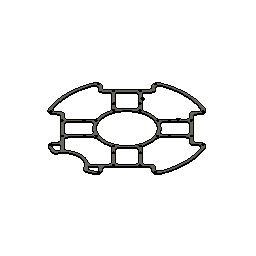
下板 v13 (Autodesk Fusion 360 design; units mm, degrees)
Autodesk Fusion 360 part; units mm, degrees
note: some values were not read from the file. Chosen so that the rebuilt part matches the saved one: which face or edge a step refers to; which pieces of a blend or face edit are solid. Set by a fixed rule: which sketch regions a step uses.
(part 1 of 5)
sketch "スケッチ1" plane through (0, 0, 0) normal (0, 0, 1) x (1, 0, 0)
  line L0 (-58.124, 63.7809) -> (-63.7809, 58.124)
  line L1 (-47.1639, 91.0045) -> (-40.8846, 84.7252)
  circle A0 centre (-62.3667, 62.3667) radius 1
  line L2 (-65.9022, 67.3164) -> (-70.852, 72.2662)
  line L3 (-35.8502, 54.9421) -> (-44.3355, 63.4273)
  arc A1 (-31.9886, 75.7742) -> (-31.9974, 82.8509) centre (-35.5257, 79.3082) ccw
  line L4 (-63.7809, 58.124) -> (-62.0978, 56.4409)
  line L5 (-33.8135, 84.7252) -> (-37.0951, 88.0068)
  line L6 (-68.0235, 65.1951) -> (-62.3667, 59.5382)
  line L7 (-54.5885, 60.2454) -> (-58.124, 63.7809)
  arc A2 (-46.9055, 91.138) -> (-47.1639, 91.0045) centre (0, 0) ccw
  arc A3 (-40.8846, 77.6541) -> (-40.8846, 84.7252) centre (-44.4201, 81.1896) ccw
  line L8 (-49.7234, 68.8153) -> (-68.8153, 49.7234)
  arc A4 (-84.7252, 40.8846) -> (-77.6541, 40.8846) centre (-81.1896, 44.4201) ccw
  line L9 (-55.6492, 27.3649) -> (-37.9715, 9.6872)
  arc A5 (-82.8374, 31.9257) -> (-75.8019, 31.9609) centre (-79.3374, 35.4964) ccw
  line L10 (-49.9923, 33.0217) -> (-53.8814, 36.9108)
  arc A6 (-88.0068, 37.0951) -> (-96.2368, 35.2806) centre (-91.5424, 33.5596) ccw
  line L11 (-31.9611, 14.9905) -> (-32.3146, 15.3441)
  circle A7 centre (-49.8155, 26.1275) radius 1.75
  line L12 (-34.167, -17.1965) -> (-34.0956, -17.125)
  arc A8 (-89.7814, 45.9408) -> (-97.869, 44.4738) centre (-93.3169, 42.4052) ccw
  line L13 (-83.0899, 32.1782) -> (-81.1896, 30.278)
  circle A9 centre (-39.2089, 15.5208) radius 1.75
  line L14 (-80.8769, 30.5907) -> (-81.1896, 30.278)
  line L15 (-85.4323, 41.5917) -> (-91.0045, 47.1639)
  line L16 (-86.1394, 35.2277) -> (-82.8374, 31.9257)
  line L17 (-88.4889, 37.5772) -> (-86.1394, 35.2277)
  line L18 (-85.4323, 41.5917) -> (-84.7252, 40.8846)
  line L19 (-70.852, 72.2662) -> (-72.2662, 70.852)
  arc A10 (-96.2368, 35.2806) -> (-96.2368, -35.2806) centre (0, 0) ccw
  line L20 (-49.7234, 68.8153) -> (-68.8153, 49.7234)
  arc A11 (-35.2806, 96.2368) -> (-37.0951, 88.0068) centre (-33.5596, 91.5424) ccw
  line L21 (-49.7234, 68.8153) -> (-40.8846, 77.6541)
  line L22 (-47.1639, 91.0045) -> (-45.9408, 89.7814)
  line L23 (-72.2662, 70.852) -> (-67.3164, 65.9022)
  arc A12 (-97.869, 44.4738) -> (-97.869, -44.4738) centre (0, 0) ccw
  circle A13 centre (-26.1275, 49.8155) radius 1.75
  line L24 (-59.5382, 62.3667) -> (-65.1951, 68.0235)
  line L25 (-36.9108, 53.8814) -> (-33.0217, 49.9923)
  line L26 (-37.5772, -88.4889) -> (-35.2277, -86.1394)
  arc A14 (-40.3326, -91.2443) -> (-39.6929, -94.5025) centre (-38.9184, -92.6585) ccw
  arc A15 (-37.9256, -100.5859) -> (-37.9262, -100.5876) centre (0, -113.3) ccw
  arc A16 (-31.321, -97.5974) -> (-31.2855, -97.6087) centre (0, 0) ccw
  line L27 (-84.7252, -33.8135) -> (-88.0068, -37.0951)
  line L28 (-41.5917, -85.4323) -> (-40.8846, -84.7252)
  arc A17 (-44.4738, -97.869) -> (-37.8014, -100.6345) centre (0, 0) ccw
  line L29 (-91.0045, -47.1639) -> (-85.4323, -41.5917)
  arc A18 (-39.6929, -94.5025) -> (-37.7434, -95.2979) centre (0, 0) ccw
  arc A19 (-40.8846, -84.7252) -> (-40.8846, -77.6541) centre (-44.4201, -81.1896) ccw
  arc A20 (-37.9256, -100.5859) -> (-37.9262, -100.5876) centre (0, -113.3) ccw
  arc A21 (-77.6541, -33.8135) -> (-84.7252, -33.8135) centre (-81.1896, -37.349) ccw
  line L30 (-41.5917, -85.4323) -> (-45.9408, -89.7814)
  line L31 (-91.0045, -47.1639) -> (-89.7814, -45.9408)
  arc A22 (-97.869, -44.4738) -> (-89.7814, -45.9408) centre (-93.3169, -42.4052) ccw
  circle A23 centre (-15.5208, 39.2089) radius 1.75
  line L32 (-65.1951, 68.0235) -> (-68.0235, 65.1951)
  line L33 (-69.0842, 69.0842) -> (-47.1639, 91.0045)
  line L34 (-15.3441, 32.3146) -> (-14.9905, 31.9611)
  line L35 (-91.0045, 47.1639) -> (-69.0842, 69.0842)
  line L36 (-37.9715, 9.6872) -> (-9.6872, 37.9715)
  line L37 (-27.3649, 55.6492) -> (-55.6492, 27.3649)
  line L38 (-63.4273, 44.3355) -> (-54.9421, 35.8502)
  line L39 (-62.0978, 56.4409) -> (-77.6541, 40.8846)
  arc A24 (0, 107.5) -> (-44.4738, 97.869) centre (0, 0) ccw
  line L40 (-56.4409, -62.0978) -> (-40.8846, -77.6541)
  line L41 (-54.9421, 35.8502) -> (-35.8502, 54.9421)
  arc A25 (-44.4738, 97.869) -> (-45.9408, 89.7814) centre (-42.4052, 93.3169) ccw
  line L42 (-14.9905, 31.9611) -> (-31.9611, 14.9905)
  line L43 (-9.6872, 37.9715) -> (-27.3649, 55.6492)
  arc A26 (0, 102.5) -> (-35.2806, 96.2368) centre (0, 0) ccw
  arc A27 (-77.6541, -40.8846) -> (-84.7252, -40.8846) centre (-81.1896, -44.4201) ccw
  arc A28 (-31.321, -97.5974) -> (-31.2855, -97.6087) centre (0, 0) ccw
  line L44 (-56.4409, -62.0978) -> (-62.0978, -56.4409)
  line L45 (-68.8153, -49.7234) -> (-49.7234, -68.8153)
  line L46 (-17.125, -34.0956) -> (-17.1965, -34.167)
  line L47 (-91.0045, -47.1639) -> (-84.7252, -40.8846)
  line L48 (-56.4409, -62.0978) -> (-62.0978, -56.4409)
  arc A29 (-32.3993, -86.1394) -> (-35.2277, -86.1394) centre (-33.8135, -87.5536) ccw
  line L49 (-68.8153, -49.7234) -> (-49.7234, -68.8153)
  line L50 (-68.8153, -49.7234) -> (-77.6541, -40.8846)
  line L51 (-32.3993, -86.1394) -> (-32.0426, -86.496)
  arc A30 (-37.9256, -100.5859) -> (-37.9262, -100.5876) centre (0, -113.3) ccw
  line L52 (-37.5772, -88.4889) -> (-40.3326, -91.2443)
  arc A31 (-96.2368, -35.2806) -> (-88.0068, -37.0951) centre (-91.5424, -33.5596) ccw
  arc A32 (-45.9408, -89.7814) -> (-44.4738, -97.869) centre (-42.4052, -93.3169) ccw
  arc A33 (-37.9256, -100.5859) -> (-37.8014, -100.6345) centre (-36.0432, -95.9538) ccw
  line L53 (-30.5907, -80.8769) -> (-21.5579, -89.9097)
  line L54 (-32.0426, -86.496) -> (-26.1835, -92.3551)
  line L55 (-37.7434, -95.2979) -> (-37.7266, -95.3045)
  line L56 (-23.7812, -100.8277) -> (-23.7402, -100.844)
  arc A34 (-43.0296, -15.8059) -> (-41.7301, -10.9963) centre (-46.5651, -12.2704) ccw
  arc A35 (-41.7301, 10.9963) -> (-41.7301, -10.9963) centre (0, 0) ccw
  line L57 (-62.6322, 42.4797) -> (-43.4926, 23.3401)
  arc A36 (-24.0851, 35.8083) -> (-35.8083, 24.0851) centre (0, 0) ccw
  arc A37 (-24.0851, 35.8083) -> (-35.8083, 24.0851) centre (0, 0) ccw
  arc A38 (0, 43.1547) -> (-10.9963, 41.7301) centre (0, 0) ccw
  arc A39 (0, 43.1547) -> (-10.9963, 41.7301) centre (0, 0) ccw
  arc A40 (-24.0851, 35.8083) -> (-35.8083, 24.0851) centre (0, 0) ccw
  arc A41 (-24.0851, 35.8083) -> (-23.3401, 43.4926) centre (-26.8756, 39.9571) ccw
  arc A42 (0, 43.1547) -> (-10.9963, 41.7301) centre (0, 0) ccw
  arc A43 (-24.0851, 35.8083) -> (-23.3401, 43.4926) centre (-26.8756, 39.9571) ccw
  arc A44 (-43.0296, -15.8059) -> (-41.7301, -10.9963) centre (-46.5651, -12.2704) ccw
  line L58 (-66.1678, 38.9441) -> (-43.0296, 15.8059)
  line L59 (-62.6322, 42.4797) -> (-43.4926, 23.3401)
  arc A45 (-41.7301, 10.9963) -> (-43.0296, 15.8059) centre (-46.5651, 12.2704) ccw
  line L60 (-66.1678, 38.9441) -> (-43.0296, 15.8059)
  arc A46 (-15.8059, 43.0296) -> (-10.9963, 41.7301) centre (-12.2704, 46.5651) ccw
  arc A47 (-15.8059, 43.0296) -> (-10.9963, 41.7301) centre (-12.2704, 46.5651) ccw
  arc A48 (-43.4926, 23.3401) -> (-35.8083, 24.0851) centre (-39.9571, 26.8756) ccw
  arc A49 (-43.4926, 23.3401) -> (-35.8083, 24.0851) centre (-39.9571, 26.8756) ccw
  arc A50 (-41.7301, 10.9963) -> (-41.7301, -10.9963) centre (0, 0) ccw
  arc A51 (-41.7301, 10.9963) -> (-41.7301, -10.9963) centre (0, 0) ccw
  arc A52 (-41.7301, 10.9963) -> (-43.0296, 15.8059) centre (-46.5651, 12.2704) ccw
  arc A53 (-10.9963, -41.7301) -> (-15.8059, -43.0296) centre (-12.2704, -46.5651) ccw
  line L61 (-38.9441, 66.1678) -> (-15.8059, 43.0296)
  arc A54 (-35.8083, -24.0851) -> (-24.0851, -35.8083) centre (0, 0) ccw
  arc A55 (-35.8083, -24.0851) -> (-43.4926, -23.3401) centre (-39.9571, -26.8756) ccw
  arc A56 (-10.9963, -41.7301) -> (-15.8059, -43.0296) centre (-12.2704, -46.5651) ccw
  line L62 (-42.4797, 62.6322) -> (-23.3401, 43.4926)
  line L63 (-42.4797, 62.6322) -> (-23.3401, 43.4926)
  arc A57 (-35.8083, -24.0851) -> (-24.0851, -35.8083) centre (0, 0) ccw
  line L64 (-62.6322, -42.4797) -> (-43.4926, -23.3401)
  arc A58 (-10.9963, -41.7301) -> (0, -43.1547) centre (0, 0) ccw
  arc A59 (-23.3401, -43.4926) -> (-24.0851, -35.8083) centre (-26.8756, -39.9571) ccw
  arc A60 (-10.9963, -41.7301) -> (0, -43.1547) centre (0, 0) ccw
  line L65 (-38.9441, 66.1678) -> (-15.8059, 43.0296)
  arc A61 (-35.8083, -24.0851) -> (-24.0851, -35.8083) centre (0, 0) ccw
  line L66 (-62.6322, -42.4797) -> (-43.4926, -23.3401)
  line L67 (-38.9441, -66.1678) -> (-15.8059, -43.0296)
  line L68 (-38.9441, -66.1678) -> (-29.7476, -56.9712)
  line L69 (-66.1678, -38.9441) -> (-43.0296, -15.8059)
  arc A62 (-29.5575, -103.3567) -> (-23.7528, -100.868) centre (-28.1827, -98.5494) ccw
  line L70 (-42.4797, -62.6322) -> (-23.3401, -43.4926)
  line L71 (-66.1678, -38.9441) -> (-43.0296, -15.8059)
  arc A63 (0, -86.4905) -> (-23.7528, -100.868) centre (0, -113.3) ccw
  arc A64 (-39.6929, -94.5025) -> (-32.0144, -97.3721) centre (0, 0) ccw
  arc A65 (-39.6929, -94.5025) -> (-32.0144, -97.3721) centre (0, 0) ccw
  arc A66 (-44.4738, -97.869) -> (-29.5575, -103.3567) centre (0, 0) ccw
  line L72 (-42.4797, -62.6322) -> (-23.3401, -43.4926)
  arc A67 (0, 38.1547) -> (0, -38.1547) centre (0, 0) ccw
  arc A68 (-44.4738, -97.869) -> (-29.5575, -103.3567) centre (0, 0) ccw
  arc A69 (-32.0144, -97.3721) -> (-26.3162, -95.431) centre (-30.4528, -92.6222) ccw
  arc A70 (0, -86.4905) -> (-23.7528, -100.868) centre (0, -113.3) ccw
  arc A71 (0, 38.1547) -> (0, -38.1547) centre (0, 0) ccw
  arc A72 (0, -81.4905) -> (-21.5579, -89.9097) centre (0, -113.3) ccw
  arc A73 (-25.9652, -94.9247) -> (-26.3162, -95.431) centre (0, -113.3) ccw
  arc A74 (0, -81.4905) -> (-21.5579, -89.9097) centre (0, -113.3) ccw
  arc A75 (-25.9652, -94.9247) -> (-26.3162, -95.431) centre (0, -113.3) ccw
  line L73 (-62.6322, 42.4797) -> (-63.9577, 43.8051)
  line L74 (-66.1678, 38.9441) -> (-67.4932, 40.2696)
  line L75 (-42.4797, 62.6322) -> (-43.8051, 63.9577)
  line L76 (-38.9441, 66.1678) -> (-40.2696, 67.4932)
  line L77 (-62.6322, -42.4797) -> (-65.8101, -45.6575)
  line L78 (-66.1678, -38.9441) -> (-69.3456, -42.122)
  line L79 (-42.4797, -62.6322) -> (-45.6575, -65.8101)
  line L80 (-38.9441, -66.1678) -> (-42.122, -69.3456)
  line L81 (-75.8019, 31.9609) -> (-67.4932, 40.2696)
  line L82 (-63.9577, 43.8051) -> (-43.8051, 63.9577)
  line L83 (-40.2696, 67.4932) -> (-31.9886, 75.7742)
  line L84 (-69.3456, -42.122) -> (-77.6541, -33.8135)
  line L85 (-30.5907, -80.8769) -> (-42.122, -69.3456)
  line L86 (-45.6575, -65.8101) -> (-65.8101, -45.6575)
  arc A76 (-25.9652, -94.9247) -> (-26.1835, -92.3551) centre (-27.5978, -93.7693) ccw
  circle A77 centre (-91.0045, 47.1639) radius 0.5
  arc A78 (0, 102.5) -> (0, -102.5) centre (0, 0) ccw
  line L87 (-17.1965, -34.167) -> (-17.4152, -33.9483)
  line L88 (-33.9483, -17.4152) -> (-34.167, -17.1965)
  line L89 (-17.1965, -34.167) -> (-17.4152, -33.9483)
  line L90 (-33.9483, -17.4152) -> (-34.167, -17.1965)
  line L91 (-17.1965, -34.167) -> (-17.4152, -33.9483)
  line L92 (-33.9483, -17.4152) -> (-34.167, -17.1965)
  line L93 (-69.0842, -69.0842) -> (-91.0045, -47.1639)
  line L94 (-47.1639, -91.0045) -> (-69.0842, -69.0842)
  line L95 (-67.3164, -65.9022) -> (-72.2662, -70.852)
  line L96 (-70.852, -72.2662) -> (-65.9022, -67.3164)
  line L97 (-72.2662, -70.852) -> (-70.852, -72.2662)
  line L98 (-68.0235, -65.1951) -> (-65.1951, -68.0235)
  line L99 (-62.3667, -59.5382) -> (-68.0235, -65.1951)
  line L100 (-65.1951, -68.0235) -> (-59.5382, -62.3667)
  circle A79 centre (-62.3667, -62.3667) radius 1
  line L101 (-63.7809, -58.124) -> (-58.124, -63.7809)
  line L102 (-58.124, -63.7809) -> (-56.4409, -62.0978)
  line L103 (-60.2454, -54.5885) -> (-63.7809, -58.124)
  line L104 (-44.3355, -63.4273) -> (-35.8502, -54.9421)
  line L105 (-54.9421, -35.8502) -> (-63.4273, -44.3355)
  line L106 (-35.8502, -54.9421) -> (-54.9421, -35.8502)
  line L107 (-53.8814, -36.9108) -> (-49.9923, -33.0217)
  line L108 (-33.0217, -49.9923) -> (-36.9108, -53.8814)
  line L109 (-55.6492, -27.3649) -> (-27.3649, -55.6492)
  circle A80 centre (-49.8155, -26.1275) radius 1.75
  circle A81 centre (-39.2089, -15.5208) radius 1.75
  circle A82 centre (-15.5208, -39.2089) radius 1.75
  circle A83 centre (-26.1275, -49.8155) radius 1.75
  line L110 (-27.3649, -55.6492) -> (-9.6872, -37.9715)
  line L111 (-9.6872, -37.9715) -> (-37.9715, -9.6872)
  line L112 (-31.9611, -14.9905) -> (-14.9905, -31.9611)
  line L113 (-37.9715, -9.6872) -> (-55.6492, -27.3649)
  line L114 (-14.9905, -31.9611) -> (-15.3441, -32.3146)
  line L115 (-32.3146, -15.3441) -> (-31.9611, -14.9905)
  arc A84 (0, -102.5) -> (0, 102.5) centre (0, 0) ccw
  line L116 (68.0235, -65.1951) -> (65.1951, -68.0235)
  line L117 (91.0045, -47.1639) -> (89.7814, -45.9408)
  arc A85 (41.7301, -10.9963) -> (41.7301, 10.9963) centre (0, 0) ccw
  line L118 (66.1678, -38.9441) -> (69.3456, -42.122)
  arc A86 (88.0068, -37.0951) -> (96.2368, -35.2806) centre (91.5424, -33.5596) ccw
  arc A87 (41.7301, -10.9963) -> (41.7301, 10.9963) centre (0, 0) ccw
  line L119 (69.3456, -42.122) -> (77.6541, -33.8135)
  arc A88 (84.7252, -40.8846) -> (77.6541, -40.8846) centre (81.1896, -44.4201) ccw
  line L120 (91.0045, -47.1639) -> (84.7252, -40.8846)
  line L121 (62.3667, -59.5382) -> (68.0235, -65.1951)
  line L122 (70.852, -72.2662) -> (65.9022, -67.3164)
  arc A89 (96.2368, -35.2806) -> (96.2368, 35.2806) centre (0, 0) ccw
  line L123 (65.1951, -68.0235) -> (59.5382, -62.3667)
  circle A90 centre (62.3667, -62.3667) radius 1
  line L124 (0, 107.5) -> (0, -102.5)
  line L125 (63.7809, -58.124) -> (58.124, -63.7809)
  line L126 (69.0842, -69.0842) -> (91.0045, -47.1639)
  line L127 (67.3164, -65.9022) -> (72.2662, -70.852)
  line L128 (58.124, -63.7809) -> (56.4409, -62.0978)
  line L129 (72.2662, -70.852) -> (70.852, -72.2662)
  line L130 (68.8153, -49.7234) -> (49.7234, -68.8153)
  line L131 (49.7234, 68.8153) -> (68.8153, 49.7234)
  line L132 (35.8502, -54.9421) -> (54.9421, -35.8502)
  line L133 (45.6575, -65.8101) -> (65.8101, -45.6575)
  arc A91 (10.9963, 41.7301) -> (0, 43.1547) centre (0, 0) ccw
  line L134 (56.4409, -62.0978) -> (40.8846, -77.6541)
  line L135 (66.1678, -38.9441) -> (43.0296, -15.8059)
  line L136 (62.6322, -42.4797) -> (43.4926, -23.3401)
  arc A92 (24.0851, -35.8083) -> (23.3401, -43.4926) centre (26.8756, -39.9571) ccw
  arc A93 (10.9963, 41.7301) -> (0, 43.1547) centre (0, 0) ccw
  arc A94 (35.2806, 96.2368) -> (0, 102.5) centre (0, 0) ccw
  arc A95 (15.8059, -43.0296) -> (10.9963, -41.7301) centre (12.2704, -46.5651) ccw
  line L137 (68.8153, -49.7234) -> (49.7234, -68.8153)
  line L138 (66.1678, -38.9441) -> (43.0296, -15.8059)
  line L139 (63.9577, 43.8051) -> (43.8051, 63.9577)
  arc A96 (0, -43.1547) -> (10.9963, -41.7301) centre (0, 0) ccw
  line L140 (91.0045, 47.1639) -> (69.0842, 69.0842)
  arc A97 (15.8059, -43.0296) -> (10.9963, -41.7301) centre (12.2704, -46.5651) ccw
  arc A98 (10.9963, 41.7301) -> (0, 43.1547) centre (0, 0) ccw
  line L141 (42.4797, 62.6322) -> (23.3401, 43.4926)
  arc A99 (0, -43.1547) -> (10.9963, -41.7301) centre (0, 0) ccw
  arc A100 (44.4738, 97.869) -> (0, 107.5) centre (0, 0) ccw
  line L142 (62.6322, -42.4797) -> (43.4926, -23.3401)
  line L143 (27.3649, -55.6492) -> (9.6872, -37.9715)
  line L144 (62.0978, 56.4409) -> (77.6541, 40.8846)
  line L145 (54.9421, 35.8502) -> (35.8502, 54.9421)
  line L146 (38.9441, 66.1678) -> (15.8059, 43.0296)
  circle A101 centre (26.1275, 49.8155) radius 1.75
  line L147 (49.7234, 68.8153) -> (68.8153, 49.7234)
  circle A102 centre (26.1275, -49.8155) radius 1.75
  arc A103 (97.869, -44.4738) -> (97.869, 44.4738) centre (0, 0) ccw
  line L148 (33.0217, -49.9923) -> (36.9108, -53.8814)
  circle A104 centre (15.5208, -39.2089) radius 1.75
  line L149 (54.9421, -35.8502) -> (63.4273, -44.3355)
  line L150 (68.8153, -49.7234) -> (77.6541, -40.8846)
  line L151 (60.2454, -54.5885) -> (63.7809, -58.124)
  line L152 (56.4409, -62.0978) -> (62.0978, -56.4409)
  line L153 (56.4409, -62.0978) -> (62.0978, -56.4409)
  arc A105 (41.7301, -10.9963) -> (41.7301, 10.9963) centre (0, 0) ccw
  arc A106 (89.7814, -45.9408) -> (97.869, -44.4738) centre (93.3169, -42.4052) ccw
  line L154 (84.7252, -33.8135) -> (88.0068, -37.0951)
  line L155 (91.0045, -47.1639) -> (85.4323, -41.5917)
  arc A107 (84.7252, -33.8135) -> (77.6541, -33.8135) centre (81.1896, -37.349) ccw
  arc A108 (0, -38.1547) -> (0, 38.1547) centre (0, 0) ccw
  line L156 (62.6322, -42.4797) -> (65.8101, -45.6575)
  line L157 (42.4797, 62.6322) -> (23.3401, 43.4926)
  line L158 (36.9108, 53.8814) -> (33.0217, 49.9923)
  line L159 (75.8019, 31.9609) -> (67.4932, 40.2696)
  line L160 (17.1965, -34.167) -> (17.4152, -33.9483)
  line L161 (53.8814, -36.9108) -> (49.9923, -33.0217)
  arc A109 (24.0851, -35.8083) -> (35.8083, -24.0851) centre (0, 0) ccw
  line L162 (17.1965, -34.167) -> (17.4152, -33.9483)
  line L163 (85.4323, 41.5917) -> (91.0045, 47.1639)
  line L164 (38.9441, 66.1678) -> (40.2696, 67.4932)
  line L165 (55.6492, -27.3649) -> (27.3649, -55.6492)
  line L166 (27.3649, 55.6492) -> (55.6492, 27.3649)
  line L167 (42.4797, -62.6322) -> (23.3401, -43.4926)
  line L168 (66.1678, 38.9441) -> (43.0296, 15.8059)
  line L169 (38.9441, 66.1678) -> (15.8059, 43.0296)
  line L170 (32.3146, -15.3441) -> (31.9611, -14.9905)
  line L171 (33.9483, -17.4152) -> (34.167, -17.1965)
  line L172 (55.6492, 27.3649) -> (37.9715, 9.6872)
  line L173 (33.9483, -17.4152) -> (34.167, -17.1965)
  line L174 (17.1965, -34.167) -> (17.4152, -33.9483)
  line L175 (40.2696, 67.4932) -> (31.9886, 75.7742)
  arc A110 (24.0851, -35.8083) -> (35.8083, -24.0851) centre (0, 0) ccw
  line L176 (35.8502, 54.9421) -> (44.3355, 63.4273)
  line L177 (62.6322, 42.4797) -> (43.4926, 23.3401)
  line L178 (62.6322, 42.4797) -> (43.4926, 23.3401)
  circle A111 centre (39.2089, 15.5208) radius 1.75
  line L179 (85.4323, 41.5917) -> (84.7252, 40.8846)
  line L180 (34.167, -17.1965) -> (34.0956, -17.125)
  line L181 (54.5885, 60.2454) -> (58.124, 63.7809)
  line L182 (37.9715, -9.6872) -> (55.6492, -27.3649)
  line L183 (47.1639, -91.0045) -> (69.0842, -69.0842)
  circle A112 centre (49.8155, -26.1275) radius 1.75
  line L184 (14.9905, -31.9611) -> (15.3441, -32.3146)
  line L185 (38.9441, -66.1678) -> (15.8059, -43.0296)
  line L186 (9.6872, 37.9715) -> (27.3649, 55.6492)
  arc A113 (96.2368, 35.2806) -> (88.0068, 37.0951) centre (91.5424, 33.5596) ccw
  arc A114 (23.7528, -100.868) -> (29.5575, -103.3567) centre (28.1827, -98.5494) ccw
  line L187 (86.1394, 35.2277) -> (82.8374, 31.9257)
  line L188 (49.9923, 33.0217) -> (53.8814, 36.9108)
  line L189 (38.9441, -66.1678) -> (29.7476, -56.9712)
  line L190 (42.4797, -62.6322) -> (23.3401, -43.4926)
  arc A115 (24.0851, -35.8083) -> (35.8083, -24.0851) centre (0, 0) ccw
  circle A116 centre (39.2089, -15.5208) radius 1.75
  line L191 (31.9611, -14.9905) -> (14.9905, -31.9611)
  line L192 (62.6322, 42.4797) -> (63.9577, 43.8051)
  line L193 (49.7234, 68.8153) -> (40.8846, 77.6541)
  line L194 (83.0899, 32.1782) -> (81.1896, 30.278)
  line L195 (44.3355, -63.4273) -> (35.8502, -54.9421)
  line L196 (66.1678, 38.9441) -> (43.0296, 15.8059)
  arc A117 (35.8083, 24.0851) -> (43.4926, 23.3401) centre (39.9571, 26.8756) ccw
  line L197 (30.5907, -80.8769) -> (21.5579, -89.9097)
  line L198 (9.6872, -37.9715) -> (37.9715, -9.6872)
  line L199 (15.3441, 32.3146) -> (14.9905, 31.9611)
  line L200 (88.4889, 37.5772) -> (86.1394, 35.2277)
  line L201 (17.125, -34.0956) -> (17.1965, -34.167)
  arc A118 (41.7301, -10.9963) -> (43.0296, -15.8059) centre (46.5651, -12.2704) ccw
  line L202 (80.8769, 30.5907) -> (81.1896, 30.278)
  arc A119 (26.3162, -95.431) -> (32.0144, -97.3721) centre (30.4528, -92.6222) ccw
  line L203 (32.0426, -86.496) -> (26.1835, -92.3551)
  circle A120 centre (91.0045, 47.1639) radius 0.5
  arc A121 (77.6541, 40.8846) -> (84.7252, 40.8846) centre (81.1896, 44.4201) ccw
  line L204 (63.7809, 58.124) -> (62.0978, 56.4409)
  circle A122 centre (49.8155, 26.1275) radius 1.75
  line L205 (66.1678, 38.9441) -> (67.4932, 40.2696)
  arc A123 (43.0296, 15.8059) -> (41.7301, 10.9963) centre (46.5651, 12.2704) ccw
  line L206 (65.1951, 68.0235) -> (68.0235, 65.1951)
  arc A124 (29.5575, -103.3567) -> (44.4738, -97.869) centre (0, 0) ccw
  line L207 (47.1639, 91.0045) -> (40.8846, 84.7252)
  line L208 (37.5772, -88.4889) -> (35.2277, -86.1394)
  arc A125 (35.8083, 24.0851) -> (24.0851, 35.8083) centre (0, 0) ccw
  arc A126 (37.8014, -100.6345) -> (44.4738, -97.869) centre (0, 0) ccw
  arc A127 (10.9963, 41.7301) -> (15.8059, 43.0296) centre (12.2704, 46.5651) ccw
  arc A128 (23.7528, -100.868) -> (0, -86.4905) centre (0, -113.3) ccw
  arc A129 (10.9963, 41.7301) -> (15.8059, 43.0296) centre (12.2704, 46.5651) ccw
  arc A130 (75.8019, 31.9609) -> (82.8374, 31.9257) centre (79.3374, 35.4964) ccw
  arc A131 (43.0296, 15.8059) -> (41.7301, 10.9963) centre (46.5651, 12.2704) ccw
  arc A132 (23.3401, 43.4926) -> (24.0851, 35.8083) centre (26.8756, 39.9571) ccw
  arc A133 (32.0144, -97.3721) -> (39.6929, -94.5025) centre (0, 0) ccw
  line L209 (33.9483, -17.4152) -> (34.167, -17.1965)
  arc A134 (41.7301, -10.9963) -> (43.0296, -15.8059) centre (46.5651, -12.2704) ccw
  line L210 (69.0842, 69.0842) -> (47.1639, 91.0045)
  line L211 (23.7812, -100.8277) -> (23.7402, -100.844)
  arc A135 (35.8083, 24.0851) -> (24.0851, 35.8083) centre (0, 0) ccw
  arc A136 (40.8846, 84.7252) -> (40.8846, 77.6541) centre (44.4201, 81.1896) ccw
  arc A137 (45.9408, 89.7814) -> (44.4738, 97.869) centre (42.4052, 93.3169) ccw
  arc A138 (31.2855, -97.6087) -> (31.321, -97.5974) centre (0, 0) ccw
  line L212 (68.0235, 65.1951) -> (62.3667, 59.5382)
  line L213 (41.5917, -85.4323) -> (40.8846, -84.7252)
  arc A139 (23.7528, -100.868) -> (0, -86.4905) centre (0, -113.3) ccw
  line L214 (31.9611, 14.9905) -> (32.3146, 15.3441)
  arc A140 (37.9262, -100.5876) -> (37.9256, -100.5859) centre (0, -113.3) ccw
  circle A141 centre (15.5208, 39.2089) radius 1.75
  line L215 (30.5907, -80.8769) -> (42.122, -69.3456)
  arc A142 (21.5579, -89.9097) -> (0, -81.4905) centre (0, -113.3) ccw
  line L216 (14.9905, 31.9611) -> (31.9611, 14.9905)
  line L217 (41.5917, -85.4323) -> (45.9408, -89.7814)
  arc A143 (43.4926, -23.3401) -> (35.8083, -24.0851) centre (39.9571, -26.8756) ccw
  arc A144 (35.8083, 24.0851) -> (24.0851, 35.8083) centre (0, 0) ccw
  arc A145 (97.869, 44.4738) -> (89.7814, 45.9408) centre (93.3169, 42.4052) ccw
  line L218 (63.4273, 44.3355) -> (54.9421, 35.8502)
  arc A146 (35.2277, -86.1394) -> (32.3993, -86.1394) centre (33.8135, -87.5536) ccw
  line L219 (65.9022, 67.3164) -> (70.852, 72.2662)
  arc A147 (21.5579, -89.9097) -> (0, -81.4905) centre (0, -113.3) ccw
  line L220 (42.4797, 62.6322) -> (43.8051, 63.9577)
  arc A148 (31.9974, 82.8509) -> (31.9886, 75.7742) centre (35.5257, 79.3082) ccw
  line L221 (32.3993, -86.1394) -> (32.0426, -86.496)
  line L222 (72.2662, 70.852) -> (67.3164, 65.9022)
  arc A149 (29.5575, -103.3567) -> (44.4738, -97.869) centre (0, 0) ccw
  arc A150 (23.3401, 43.4926) -> (24.0851, 35.8083) centre (26.8756, 39.9571) ccw
  arc A151 (47.1639, 91.0045) -> (46.9055, 91.138) centre (0, 0) ccw
  arc A152 (39.6929, -94.5025) -> (40.3326, -91.2443) centre (38.9184, -92.6585) ccw
  arc A153 (35.8083, 24.0851) -> (43.4926, 23.3401) centre (39.9571, 26.8756) ccw
  line L223 (37.9715, 9.6872) -> (9.6872, 37.9715)
  arc A154 (37.9262, -100.5876) -> (37.9256, -100.5859) centre (0, -113.3) ccw
  arc A155 (26.1835, -92.3551) -> (25.9652, -94.9247) centre (27.5978, -93.7693) ccw
  arc A156 (37.8014, -100.6345) -> (37.9256, -100.5859) centre (36.0432, -95.9538) ccw
  line L224 (47.1639, 91.0045) -> (45.9408, 89.7814)
  line L225 (70.852, 72.2662) -> (72.2662, 70.852)
  arc A157 (37.9262, -100.5876) -> (37.9256, -100.5859) centre (0, -113.3) ccw
  line L226 (58.124, 63.7809) -> (63.7809, 58.124)
  line L227 (42.4797, -62.6322) -> (45.6575, -65.8101)
  circle A158 centre (62.3667, 62.3667) radius 1
  line L228 (37.7434, -95.2979) -> (37.7266, -95.3045)
  arc A159 (40.8846, -77.6541) -> (40.8846, -84.7252) centre (44.4201, -81.1896) ccw
  arc A160 (37.7434, -95.2979) -> (39.6929, -94.5025) centre (0, 0) ccw
  arc A161 (26.3162, -95.431) -> (25.9652, -94.9247) centre (0, -113.3) ccw
  arc A162 (37.0951, 88.0068) -> (35.2806, 96.2368) centre (33.5596, 91.5424) ccw
  arc A163 (26.3162, -95.431) -> (25.9652, -94.9247) centre (0, -113.3) ccw
  arc A164 (32.0144, -97.3721) -> (39.6929, -94.5025) centre (0, 0) ccw
  arc A165 (31.2855, -97.6087) -> (31.321, -97.5974) centre (0, 0) ccw
  line L229 (59.5382, 62.3667) -> (65.1951, 68.0235)
  line L230 (33.8135, 84.7252) -> (37.0951, 88.0068)
  arc A166 (44.4738, -97.869) -> (45.9408, -89.7814) centre (42.4052, -93.3169) ccw
  line L231 (38.9441, -66.1678) -> (42.122, -69.3456)
  line L232 (37.5772, -88.4889) -> (40.3326, -91.2443)
  arc A167 (0, -38.1547) -> (0, 38.1547) centre (0, 0) ccw
  line L233 (0, 107.5) -> (0, -86.4905)
  line L234 (-33.8135, 84.7252) -> (-31.9974, 82.8509)
  line L235 (33.8135, 84.7252) -> (31.9974, 82.8509)
  point P0 (-63.8655, -63.8655)
  point P1 (-81.1896, -37.349)
  point P2 (-63.8655, -63.8655)
  point P3 (-63.8655, -63.8655)
  point P4 (-37.349, 81.1896)
  point P5 (-12.2704, -46.5651)
  point P6 (-12.2704, 46.5651)
  point P7 (12.2704, -46.5651)
  point P8 (12.2704, 46.5651)
  point P9 (63.8655, -63.8655)
  point P10 (63.8655, -63.8655)
  point P11 (63.8655, -63.8655)
  point P12 (81.1896, -37.349)
  point P13 (12.2704, -46.5651)
  point P14 (37.349, 81.1896)
  point P15 (12.2704, 46.5651)
  point P16 (-12.2704, -46.5651)
  point P17 (-12.2704, 46.5651)
  dimension "d45" = 5
  dimension "d46" = 5
  dimension "d47" = 2
  dimension "d52" = 1
  constraint parallel L53 L85
  constraint tangent A18 L55
  constraint parallel L55 L56
  constraint coincident L58.end A45.end
  constraint coincident A46.start A47.start
  constraint coincident A34.start A44.start
  constraint coincident A53.end A56.end
  constraint coincident L57.end L59.end
  constraint coincident A41.end A43.end
  constraint coincident A55.end L64.end
  constraint coincident A59.start L70.end
  constraint coincident L58.end A45
  constraint coincident L57.end A48
  constraint coincident A41.end A43
  constraint coincident A47.start A46
  constraint coincident L58.end A52
  constraint coincident L57.end A49
  constraint coincident A43.end A41
  constraint coincident A46.start A47
  constraint tangent A69 A72
  constraint tangent A62 A70
  constraint concentric A36 A67
  constraint coincident A53.start A36
  constraint concentric A36 A50
  constraint concentric A50 A57
  constraint concentric A57 A58
  constraint coincident A63 L56.end
  constraint coincident A64 L55.end
  constraint concentric A72 A73
  constraint concentric A74 A75
  constraint perpendicular L73 L81
  constraint perpendicular L74 L81
  constraint perpendicular L75 L81
  constraint perpendicular L76 L81
  constraint perpendicular L77 L85
  constraint perpendicular L78 L85
  constraint perpendicular L79 L85
  constraint perpendicular L80 L85
  constraint collinear L81 L82
  constraint collinear L82 L83
  constraint collinear L84 L85
  constraint coincident L79.end L85
  constraint collinear L85 L86
  constraint coincident L82 L38.start
  constraint coincident L82 L3.end
  constraint tangent L54 A76
  constraint tangent A75 A76
  constraint coincident L15 L35.start
  constraint coincident L15.end A78
  constraint coincident A67 L87.end
  constraint coincident A67 L88.start
  constraint collinear L87 L88
  constraint collinear L89 L90
  constraint collinear L91 L92
  constraint coincident A67 L12.end
  constraint coincident A67 L46.start
  constraint coincident A78 L29.start
  measures "d45" radius of A69
  measures "d46" radius of A62
  measures "d47" radius of A76
  measures "d52" diameter of A77
extrude "押し出し1" add sketch "スケッチ1" along normal blind 1.5 contours L36 L43 A38 A39 A42 A46 A47 A67 A71 L124 L233 | L9 L36 L37 L43 L57 A36 A37 A40 A41 A43 L58 L59 A45 L60 A46 A47 A48 A49 A52 L61 L62 L63 L65 A67 A71 | A53 A56 A58 A60 A67 A71 L110 L111 L124 L233 | L9 L36 A34 A35 A44 A45 A50 A51 A52 A67 A71 L111 L113 | L12 L46 A34 A44 A53 A54 A55 A56 A57 L64 A59 A61 L66 L67 L69 L70 L71 L72 A67 A71 L87 L88 L89 L90 L91 L92 L109 L110 L111 L113 | A80 | A81 | A82 | A83 makes body 1
fillet "フィレット1" [no effect]
extrude "押し出し2" add sketch "スケッチ1" along normal blind 1.5 contours A24 A25 A26 A78 L124 L233 | A8 A10 A12 A22 A77 A78 | A84 L124 A94 A100 A137 L233 | L124 A91 A93 A98 A108 L186 A127 A129 L223 A167 L233 | L26 A14 A15 L27 L28 L29 A19 A20 A21 L30 A22 L40 A27 L44 L45 L47 L48 A29 L49 L50 L51 A30 L52 A31 A32 L53 L54 L64 L66 L67 L68 L69 L70 L71 L72 L77 L78 L79 L80 L84 L85 L86 A78 L109 A140 A154 A157 | L124 A95 A96 A97 A99 L143 A108 L198 A167 L233 | L141 L146 A108 L157 L166 L168 L169 L172 L177 L178 L186 L196 A117 A123 A125 A127 A129 A131 A132 A135 A144 A150 A153 L223 A167 | L135 L136 A92 A95 L138 A97 L142 L143 A108 L160 A109 L162 L165 L167 L171 L173 L174 A110 L180 L182 L185 L190 A115 L198 L201 A118 L209 A134 A143 A167 | A85 A87 A105 A108 L172 L182 L198 A118 A123 A131 A134 L223 A167 | A15 A17 A18 A20 A30 A32 L55 A64 A65 A66 A68 A78 A140 A154 A157 | A84 A89 A103 A106 A120 A145 | A15 A20 A30 A84 L118 A86 L119 A88 L120 L130 L133 L134 L135 L136 L137 L138 L142 L150 L152 L153 A106 L154 L155 A107 L156 L165 L167 L185 L189 L190 L197 L203 L208 L213 A140 L215 L217 A146 L221 A152 A154 A157 L227 A159 A166 L231 L232 | A15 A20 A30 A84 L124 L197 A119 L203 A128 A138 A139 A140 A142 A147 A154 A155 A157 A161 A163 A165 L233 | A15 A16 A20 A28 A30 L53 L54 A63 A69 A70 A72 A73 A74 A75 A76 A78 L124 A140 A154 A157 L233 | A15 A16 A17 A20 A28 A30 A33 A62 A63 A64 A65 A66 A68 A70 A78 A140 A154 A157 | A15 A20 A30 A84 A124 A126 A133 A140 A149 A154 A157 L228 A160 A164 A166 | A15 A20 A30 A84 A114 A124 A126 A128 A133 A138 A139 A140 A149 A154 A156 A157 A164 A165 bodies 1 makes body 2 at (0, 104.0092, 0)
extrude "押し出し3" add sketch "スケッチ1" along normal blind 1.5 contours L1 A1 L5 A3 L8 A4 A5 A6 A8 L13 L15 L16 L17 L18 L20 A11 L21 L37 L39 A25 L57 L58 L59 L60 L61 L62 L63 L65 L73 L74 L75 L76 L81 L82 L83 A77 A78 L234 | A84 L131 L139 L141 L144 L146 L147 L157 L159 L163 L164 L166 L168 L169 L175 L177 L178 L179 A113 L187 L192 L193 L194 L196 L200 A120 A121 L205 L207 A130 A136 A137 A145 L220 A148 A162 L230 L235 bodies 1 2
fillet "フィレット2" radius 5 16 edges at (40.2696, 67.4932, 0.75) (-40.2696, 67.4932, 0.75) (-43.8051, 63.9577, 0.75) (-63.9577, 43.8051, 0.75) (-67.4932, 40.2696, 0.75) (-69.3456, -42.122, 0.75) (-65.8101, -45.6575, 0.75) (-45.6575, -65.8101, 0.75) (-42.122, -69.3456, 0.75) (-21.5579, -89.9097, 0.75) (21.5579, -89.9097, 0.75) (42.122, -69.3456, 0.75) (45.6575, -65.8101, 0.75) (69.3456, -42.122, 0.75) (65.8101, -45.6575, 0.75) (67.4932, 40.2696, 0.75) on bodies 1
extrude "押し出し4" cut sketch "スケッチ1" along normal blind 100 contours A80 | A81 | A82 | A83 bodies 1
sketch "スケッチ2" plane through (0, 0, 0) normal (0, 0, -1) x (1, 0, 0)
  circle A0 centre (-26.1275, 49.8155) radius 1.75
  circle A1 centre (-39.2089, 15.5208) radius 1.75
  circle A2 centre (-15.5208, 39.2089) radius 1.75
  circle A3 centre (-49.8155, 26.1275) radius 1.75
  line L0 (-38.9441, -66.1678) -> (-15.8059, -43.0296)
  arc A4 (-10.9963, -41.7301) -> (-15.8059, -43.0296) centre (-12.2704, -46.5651) ccw
  arc A5 (-10.9963, -41.7301) -> (10.9963, -41.7301) centre (0, 0) ccw
  arc A6 (15.8059, -43.0296) -> (10.9963, -41.7301) centre (12.2704, -46.5651) ccw
  line L1 (15.8059, -43.0296) -> (38.9441, -66.1678)
  arc A7 (37.51, -70.2528) -> (38.9441, -66.1678) centre (33.9744, -66.7173) ccw
  line L2 (37.51, -70.2528) -> (31.9886, -75.7742)
  arc A8 (31.9886, -75.7742) -> (31.9974, -82.8509) centre (35.5257, -79.3082) ccw
  line L3 (31.9974, -82.8509) -> (33.8135, -84.7252)
  line L4 (33.8135, -84.7252) -> (37.0951, -88.0068)
  arc A9 (35.2806, -96.2368) -> (37.0951, -88.0068) centre (33.5596, -91.5424) ccw
  arc A10 (-35.2806, -96.2368) -> (35.2806, -96.2368) centre (0, 0) ccw
  arc A11 (-37.0951, -88.0068) -> (-35.2806, -96.2368) centre (-33.5596, -91.5424) ccw
  line L5 (-37.0951, -88.0068) -> (-33.8135, -84.7252)
  line L6 (-33.8135, -84.7252) -> (-31.9974, -82.8509)
  arc A12 (-31.9974, -82.8509) -> (-31.9886, -75.7742) centre (-35.5257, -79.3082) ccw
  line L7 (-31.9886, -75.7742) -> (-37.51, -70.2528)
  arc A13 (-38.9441, -66.1678) -> (-37.51, -70.2528) centre (-33.9744, -66.7173) ccw
  line L8 (-23.3401, -43.4926) -> (-42.4797, -62.6322)
  arc A14 (-46.5647, -61.198) -> (-42.4797, -62.6322) centre (-43.0292, -57.6625) ccw
  line L9 (-46.5647, -61.198) -> (-60.4221, -47.3407)
  arc A15 (-60.4221, -40.2696) -> (-60.4221, -47.3407) centre (-56.8866, -43.8051) ccw
  line L10 (-60.4221, -40.2696) -> (-43.4926, -23.3401)
  arc A16 (-35.8083, -24.0851) -> (-43.4926, -23.3401) centre (-39.9571, -26.8756) ccw
  arc A17 (-35.8083, -24.0851) -> (-24.0851, -35.8083) centre (0, 0) ccw
  arc A18 (-23.3401, -43.4926) -> (-24.0851, -35.8083) centre (-26.8756, -39.9571) ccw
  line L11 (-43.0296, -15.8059) -> (-63.9577, -36.7341)
  arc A19 (-71.0287, -36.7341) -> (-63.9577, -36.7341) centre (-67.4932, -33.1985) ccw
  line L12 (-71.0287, -36.7341) -> (-75.8019, -31.9609)
  arc A20 (-75.8019, -31.9609) -> (-82.8374, -31.9257) centre (-79.3374, -35.4964) ccw
  line L13 (-82.8374, -31.9257) -> (-88.0068, -37.0951)
  arc A21 (-96.2368, -35.2806) -> (-88.0068, -37.0951) centre (-91.5424, -33.5596) ccw
  arc A22 (-96.2368, 35.2806) -> (-96.2368, -35.2806) centre (0, 0) ccw
  arc A23 (-88.0068, 37.0951) -> (-96.2368, 35.2806) centre (-91.5424, 33.5596) ccw
  line L14 (-88.0068, 37.0951) -> (-84.7252, 33.8135)
  arc A24 (-84.7252, 33.8135) -> (-77.6541, 33.8135) centre (-81.1896, 37.349) ccw
  line L15 (-77.6541, 33.8135) -> (-72.863, 38.6046)
  arc A25 (-66.1678, 38.9441) -> (-72.863, 38.6046) centre (-69.3275, 35.0691) ccw
  line L16 (-66.1678, 38.9441) -> (-43.0296, 15.8059)
  arc A26 (-41.7301, 10.9963) -> (-43.0296, 15.8059) centre (-46.5651, 12.2704) ccw
  arc A27 (-41.7301, 10.9963) -> (-41.7301, -10.9963) centre (0, 0) ccw
  arc A28 (-43.0296, -15.8059) -> (-41.7301, -10.9963) centre (-46.5651, -12.2704) ccw
  arc A29 (-90.783, -46.7156) -> (-91.4938, -47.061) centre (-91.0045, -47.1639) ccw
  arc A30 (-90.783, -46.7156) -> (-89.7814, -45.9408) centre (-93.3169, -42.4052) ccw
  line L17 (-89.7814, -45.9408) -> (-84.7252, -40.8846)
  arc A31 (-77.6541, -40.8846) -> (-84.7252, -40.8846) centre (-81.1896, -44.4201) ccw
  line L18 (-77.6541, -40.8846) -> (-40.8846, -77.6541)
  arc A32 (-40.8846, -84.7252) -> (-40.8846, -77.6541) centre (-44.4201, -81.1896) ccw
  line L19 (-40.8846, -84.7252) -> (-45.9408, -89.7814)
  arc A33 (-45.9408, -89.7814) -> (-44.4738, -97.869) centre (-42.4052, -93.3169) ccw
  arc A34 (-44.4738, -97.869) -> (44.4738, -97.869) centre (0, 0) ccw
  arc A35 (44.4738, -97.869) -> (45.9408, -89.7814) centre (42.4052, -93.3169) ccw
  line L20 (45.9408, -89.7814) -> (40.8846, -84.7252)
  arc A36 (40.8846, -77.6541) -> (40.8846, -84.7252) centre (44.4201, -81.1896) ccw
  line L21 (40.8846, -77.6541) -> (77.6541, -40.8846)
  arc A37 (84.7252, -40.8846) -> (77.6541, -40.8846) centre (81.1896, -44.4201) ccw
  line L22 (84.7252, -40.8846) -> (89.7814, -45.9408)
  arc A38 (89.7814, -45.9408) -> (90.783, -46.7156) centre (93.3169, -42.4052) ccw
  arc A39 (91.4938, -47.061) -> (90.783, -46.7156) centre (91.0045, -47.1639) ccw
  arc A40 (91.4938, -47.061) -> (97.869, -44.4738) centre (93.3169, -42.4052) ccw
  arc A41 (97.869, -44.4738) -> (97.869, 44.4738) centre (0, 0) ccw
  arc A42 (97.869, 44.4738) -> (89.7814, 45.9408) centre (93.3169, 42.4052) ccw
  line L23 (89.7814, 45.9408) -> (84.7252, 40.8846)
  arc A43 (77.6541, 40.8846) -> (84.7252, 40.8846) centre (81.1896, 44.4201) ccw
  line L24 (77.6541, 40.8846) -> (40.8846, 77.6541)
  arc A44 (40.8846, 84.7252) -> (40.8846, 77.6541) centre (44.4201, 81.1896) ccw
  line L25 (40.8846, 84.7252) -> (45.9408, 89.7814)
  arc A45 (45.9408, 89.7814) -> (44.4738, 97.869) centre (42.4052, 93.3169) ccw
  arc A46 (44.4738, 97.869) -> (37.9262, 100.5876) centre (0, 0) ccw
  arc A47 (37.9256, 100.5859) -> (37.9262, 100.5876) centre (0, 113.3) ccw
  arc A48 (37.9256, 100.5859) -> (37.8014, 100.6345) centre (36.0432, 95.9538) ccw
  arc A49 (37.8014, 100.6345) -> (29.5575, 103.3567) centre (0, 0) ccw
  arc A50 (29.5575, 103.3567) -> (23.7528, 100.868) centre (28.1827, 98.5494) ccw
  arc A51 (-23.7528, 100.868) -> (23.7528, 100.868) centre (0, 113.3) ccw
  arc A52 (-23.7528, 100.868) -> (-29.5575, 103.3567) centre (-28.1827, 98.5494) ccw
  arc A53 (-29.5575, 103.3567) -> (-37.8014, 100.6345) centre (0, 0) ccw
  arc A54 (-37.8014, 100.6345) -> (-37.9256, 100.5859) centre (-36.0432, 95.9538) ccw
  arc A55 (-37.9262, 100.5876) -> (-37.9256, 100.5859) centre (0, 113.3) ccw
  arc A56 (-37.9262, 100.5876) -> (-44.4738, 97.869) centre (0, 0) ccw
  arc A57 (-44.4738, 97.869) -> (-45.9408, 89.7814) centre (-42.4052, 93.3169) ccw
  line L26 (-45.9408, 89.7814) -> (-40.8846, 84.7252)
  arc A58 (-40.8846, 77.6541) -> (-40.8846, 84.7252) centre (-44.4201, 81.1896) ccw
  line L27 (-40.8846, 77.6541) -> (-77.6541, 40.8846)
  arc A59 (-84.7252, 40.8846) -> (-77.6541, 40.8846) centre (-81.1896, 44.4201) ccw
  line L28 (-84.7252, 40.8846) -> (-89.7814, 45.9408)
  arc A60 (-89.7814, 45.9408) -> (-97.869, 44.4738) centre (-93.3169, 42.4052) ccw
  arc A61 (-97.869, 44.4738) -> (-97.869, -44.4738) centre (0, 0) ccw
  arc A62 (-97.869, -44.4738) -> (-91.4938, -47.061) centre (-93.3169, -42.4052) ccw
  arc A63 (88.0068, -37.0951) -> (96.2368, -35.2806) centre (91.5424, -33.5596) ccw
  line L29 (88.0068, -37.0951) -> (82.8374, -31.9257)
  arc A64 (82.8374, -31.9257) -> (75.8019, -31.9609) centre (79.3374, -35.4964) ccw
  line L30 (75.8019, -31.9609) -> (71.0287, -36.7341)
  arc A65 (63.9577, -36.7341) -> (71.0287, -36.7341) centre (67.4932, -33.1985) ccw
  line L31 (63.9577, -36.7341) -> (43.0296, -15.8059)
  arc A66 (41.7301, -10.9963) -> (43.0296, -15.8059) centre (46.5651, -12.2704) ccw
  arc A67 (41.7301, -10.9963) -> (41.7301, 10.9963) centre (0, 0) ccw
  arc A68 (43.0296, 15.8059) -> (41.7301, 10.9963) centre (46.5651, 12.2704) ccw
  line L32 (43.0296, 15.8059) -> (66.1678, 38.9441)
  arc A69 (72.863, 38.6046) -> (66.1678, 38.9441) centre (69.3275, 35.0691) ccw
  line L33 (72.863, 38.6046) -> (77.6541, 33.8135)
  arc A70 (77.6541, 33.8135) -> (84.7252, 33.8135) centre (81.1896, 37.349) ccw
  line L34 (84.7252, 33.8135) -> (88.0068, 37.0951)
  arc A71 (96.2368, 35.2806) -> (88.0068, 37.0951) centre (91.5424, 33.5596) ccw
  arc A72 (96.2368, -35.2806) -> (96.2368, 35.2806) centre (0, 0) ccw
  line L35 (43.4926, -23.3401) -> (63.9577, -43.8051)
  line L36 (63.9577, -43.8051) -> (43.8051, -63.9577)
  line L37 (43.8051, -63.9577) -> (42.4797, -62.6322)
  line L38 (42.4797, -62.6322) -> (23.3401, -43.4926)
  arc A73 (24.0851, -35.8083) -> (23.3401, -43.4926) centre (26.8756, -39.9571) ccw
  arc A74 (24.0851, -35.8083) -> (35.8083, -24.0851) centre (0, 0) ccw
  arc A75 (43.4926, -23.3401) -> (35.8083, -24.0851) centre (39.9571, -26.8756) ccw
  line L39 (-43.4926, 23.3401) -> (-62.6322, 42.4797)
  arc A76 (-62.2927, 49.1749) -> (-62.6322, 42.4797) centre (-58.7571, 45.6394) ccw
  line L40 (-62.2927, 49.1749) -> (-49.1931, 62.2745)
  arc A77 (-42.122, 62.2745) -> (-49.1931, 62.2745) centre (-45.6575, 58.739) ccw
  line L41 (-42.122, 62.2745) -> (-23.3401, 43.4926)
  arc A78 (-24.0851, 35.8083) -> (-23.3401, 43.4926) centre (-26.8756, 39.9571) ccw
  arc A79 (-24.0851, 35.8083) -> (-35.8083, 24.0851) centre (0, 0) ccw
  arc A80 (-43.4926, 23.3401) -> (-35.8083, 24.0851) centre (-39.9571, 26.8756) ccw
  arc A81 (-38.5865, 72.8811) -> (-38.5865, 65.8101) centre (-35.0509, 69.3456) ccw
  line L42 (-38.5865, 72.8811) -> (-24.7285, 86.7391)
  arc A82 (-18.3143, 87.2917) -> (-24.7285, 86.7391) centre (-21.193, 83.2035) ccw
  arc A83 (-18.3143, 87.2917) -> (18.3143, 87.2917) centre (0, 113.3) ccw
  arc A84 (24.7285, 86.7391) -> (18.3143, 87.2917) centre (21.193, 83.2035) ccw
  line L43 (24.7285, 86.7391) -> (38.5865, 72.8811)
  arc A85 (38.5865, 65.8101) -> (38.5865, 72.8811) centre (35.0509, 69.3456) ccw
  line L44 (38.5865, 65.8101) -> (15.8059, 43.0296)
  arc A86 (10.9963, 41.7301) -> (15.8059, 43.0296) centre (12.2704, 46.5651) ccw
  arc A87 (10.9963, 41.7301) -> (-10.9963, 41.7301) centre (0, 0) ccw
  arc A88 (-15.8059, 43.0296) -> (-10.9963, 41.7301) centre (-12.2704, 46.5651) ccw
  line L45 (-15.8059, 43.0296) -> (-38.5865, 65.8101)
  line L46 (-35.2277, 86.1394) -> (-40.3326, 91.2443)
  arc A89 (-39.6929, 94.5025) -> (-40.3326, 91.2443) centre (-38.9184, 92.6585) ccw
  arc A90 (-32.0144, 97.3721) -> (-39.6929, 94.5025) centre (0, 0) ccw
  arc A91 (-26.3162, 95.431) -> (-32.0144, 97.3721) centre (-30.4528, 92.6222) ccw
  arc A92 (-26.3162, 95.431) -> (-25.9652, 94.9247) centre (0, 113.3) ccw
  arc A93 (-26.1835, 92.3551) -> (-25.9652, 94.9247) centre (-27.5978, 93.7693) ccw
  line L47 (-26.1835, 92.3551) -> (-32.3993, 86.1394)
  arc A94 (-35.2277, 86.1394) -> (-32.3993, 86.1394) centre (-33.8135, 87.5536) ccw
  circle A95 centre (39.2089, -15.5208) radius 1.75
  circle A96 centre (15.5208, -39.2089) radius 1.75
  circle A97 centre (39.2089, 15.5208) radius 1.75
  circle A98 centre (26.1275, -49.8155) radius 1.75
  circle A99 centre (15.5208, 39.2089) radius 1.75
  circle A100 centre (49.8155, 26.1275) radius 1.75
  circle A101 centre (49.8155, -26.1275) radius 1.75
  arc A102 (23.3401, 43.4926) -> (24.0851, 35.8083) centre (26.8756, 39.9571) ccw
  line L48 (23.3401, 43.4926) -> (42.122, 62.2745)
  arc A103 (49.1931, 62.2745) -> (42.122, 62.2745) centre (45.6575, 58.739) ccw
  line L49 (49.1931, 62.2745) -> (62.2927, 49.1749)
  arc A104 (62.6322, 42.4797) -> (62.2927, 49.1749) centre (58.7571, 45.6394) ccw
  line L50 (62.6322, 42.4797) -> (43.4926, 23.3401)
  arc A105 (35.8083, 24.0851) -> (43.4926, 23.3401) centre (39.9571, 26.8756) ccw
  arc A106 (35.8083, 24.0851) -> (24.0851, 35.8083) centre (0, 0) ccw
  circle A107 centre (26.1275, 49.8155) radius 1.75
  arc A108 (32.3993, 86.1394) -> (35.2277, 86.1394) centre (33.8135, 87.5536) ccw
  line L51 (32.3993, 86.1394) -> (26.1835, 92.3551)
  arc A109 (25.9652, 94.9247) -> (26.1835, 92.3551) centre (27.5978, 93.7693) ccw
  arc A110 (25.9652, 94.9247) -> (26.3162, 95.431) centre (0, 113.3) ccw
  arc A111 (32.0144, 97.3721) -> (26.3162, 95.431) centre (30.4528, 92.6222) ccw
  arc A112 (39.6929, 94.5025) -> (32.0144, 97.3721) centre (0, 0) ccw
  arc A113 (40.3326, 91.2443) -> (39.6929, 94.5025) centre (38.9184, 92.6585) ccw
  line L52 (40.3326, 91.2443) -> (35.2277, 86.1394)
  circle A114 centre (-49.8155, -26.1275) radius 1.75
  circle A115 centre (-26.1275, -49.8155) radius 1.75
  circle A116 centre (-15.5208, -39.2089) radius 1.75
  circle A117 centre (-39.2089, -15.5208) radius 1.75
  arc A118 (17.125, 34.0956) -> (-17.125, 34.0956) centre (0, 0) ccw
  line L53 (17.125, 34.0956) -> (17.1965, 34.167)
  line L54 (17.1965, 34.167) -> (17.4152, 33.9483)
  arc A119 (33.9483, 17.4152) -> (17.4152, 33.9483) centre (0, 0) ccw
  line L55 (33.9483, 17.4152) -> (34.167, 17.1965)
  line L56 (34.167, 17.1965) -> (34.0956, 17.125)
  arc A120 (-34.0956, 17.125) -> (34.0956, 17.125) centre (0, 0) ccw
  line L57 (-34.0956, 17.125) -> (-34.167, 17.1965)
  line L58 (-34.167, 17.1965) -> (-33.9483, 17.4152)
  arc A121 (-17.4152, 33.9483) -> (-33.9483, 17.4152) centre (0, 0) ccw
  line L59 (-17.4152, 33.9483) -> (-17.1965, 34.167)
  line L60 (-17.1965, 34.167) -> (-17.125, 34.0956)
  line L61 (-72.863, 38.6046) -> (-38.5865, 72.8811)
  line L62 (-66.1678, 38.9441) -> (-43.0296, 15.8059)
  line L63 (-62.6322, 42.4797) -> (-43.4926, 23.3401)
  line L64 (-42.122, 62.2745) -> (-23.3401, 43.4926)
  line L65 (-38.5865, 65.8101) -> (-15.8059, 43.0296)
  line L66 (-72.863, 38.6046) -> (-77.6541, 33.8135)
  line L67 (-88.0068, 37.0951) -> (-84.7252, 33.8135)
  arc A122 (-84.7263, 33.8146) -> (-77.653, 33.8146) centre (-81.1896, 37.349) ccw
  arc A123 (-65.4524, 38.2288) -> (-72.863, 38.6046) centre (-69.3275, 35.0691) ccw
  arc A124 (-62.2927, 49.1749) -> (-61.9168, 41.7643) centre (-58.7571, 45.6394) ccw
  arc A125 (-42.122, 62.2745) -> (-49.1931, 62.2745) centre (-45.6575, 58.739) ccw
  arc A126 (-38.5865, 72.8811) -> (-38.5865, 65.8101) centre (-35.0509, 69.3456) ccw
  line L68 (-55.7429, 55.7247) -> (-52.8534, 52.8352)
  line L69 (-37.1133, 87.9887) -> (-33.8316, 84.707)
  line L70 (-38.6227, 72.8449) -> (-33.8316, 77.636)
  arc A127 (-33.8327, 77.6349) -> (-33.8327, 84.7081) centre (-37.3672, 81.1715) ccw
  line L71 (-37.0951, -88.0068) -> (-33.8135, -84.7252)
  arc A128 (-33.8146, -84.7263) -> (-33.8146, -77.653) centre (-37.349, -81.1896) ccw
  line L72 (-38.6046, -72.863) -> (-33.8135, -77.6541)
  line L73 (-38.6046, -72.863) -> (-72.8811, -38.5865)
  line L74 (-72.8449, -38.6227) -> (-77.636, -33.8316)
  line L75 (-84.7081, -33.8327) -> (-84.707, -33.8316)
  arc A129 (-72.8811, -38.5865) -> (-65.8101, -38.5865) centre (-69.3456, -35.0509) ccw
  line L76 (-65.8101, -38.5865) -> (-43.0296, -15.8059)
  line L77 (-62.2745, -42.122) -> (-43.4926, -23.3401)
  arc A130 (-62.2745, -42.122) -> (-62.2745, -49.1931) centre (-58.739, -45.6575) ccw
  arc A131 (-49.1749, -62.2927) -> (-41.7643, -61.9168) centre (-45.6394, -58.7571) ccw
  arc A132 (-38.2288, -65.4524) -> (-38.6046, -72.863) centre (-35.0691, -69.3275) ccw
  line L78 (-38.9441, -66.1678) -> (-15.8059, -43.0296)
  line L79 (-42.4797, -62.6322) -> (-23.3401, -43.4926)
  arc A133 (84.7263, -33.8146) -> (84.7252, -33.8135) centre (81.1896, -37.349) ccw
  line L80 (77.653, -33.8146) -> (77.6541, -33.8135)
  line L81 (72.863, -38.6046) -> (38.5865, -72.8811)
  arc A134 (38.5865, -72.8811) -> (38.5865, -65.8101) centre (35.0509, -69.3456) ccw
  line L82 (38.5865, -65.8101) -> (15.8059, -43.0296)
  line L83 (42.122, -62.2745) -> (23.3401, -43.4926)
  arc A135 (42.122, -62.2745) -> (49.1931, -62.2745) centre (45.6575, -58.739) ccw
  arc A136 (62.2927, -49.1749) -> (61.9168, -41.7643) centre (58.7571, -45.6394) ccw
  arc A137 (65.4524, -38.2288) -> (72.863, -38.6046) centre (69.3275, -35.0691) ccw
  line L84 (66.1678, -38.9441) -> (43.0296, -15.8059)
  line L85 (62.6322, -42.4797) -> (43.4926, -23.3401)
  line L86 (37.0951, 88.0068) -> (33.8135, 84.7252)
  arc A138 (33.8146, 84.7263) -> (33.8146, 77.653) centre (37.349, 81.1896) ccw
  line L87 (38.6046, 72.863) -> (33.8135, 77.6541)
  line L88 (38.6046, 72.863) -> (72.8811, 38.5865)
  line L89 (72.8449, 38.6227) -> (77.636, 33.8316)
  arc A139 (77.6349, 33.8327) -> (84.7081, 33.8327) centre (81.1715, 37.3672) ccw
  line L90 (87.9887, 37.1133) -> (84.707, 33.8316)
  arc A140 (72.8811, 38.5865) -> (65.8101, 38.5865) centre (69.3456, 35.0509) ccw
  line L91 (65.8101, 38.5865) -> (43.0296, 15.8059)
  line L92 (62.2745, 42.122) -> (43.4926, 23.3401)
  arc A141 (62.2745, 42.122) -> (62.2745, 49.1931) centre (58.739, 45.6575) ccw
  arc A142 (49.1749, 62.2927) -> (41.7643, 61.9168) centre (45.6394, 58.7571) ccw
  arc A143 (38.2288, 65.4524) -> (38.6046, 72.863) centre (35.0691, 69.3275) ccw
  line L93 (38.9441, 66.1678) -> (15.8059, 43.0296)
  line L94 (42.4797, 62.6322) -> (23.3401, 43.4926)
  line L95 (-88.0068, -37.0951) -> (-84.7252, -33.8135)
  line L96 (-77.636, -33.8316) -> (-77.6541, -33.8135)
  arc A144 (-77.6541, -33.8135) -> (-84.7252, -33.8135) centre (-81.1896, -37.349) ccw
  line L97 (0, 0) -> (0, -10)
  line L98 (72.8449, -38.6227) -> (72.863, -38.6046)
  line L99 (88.0068, -37.0951) -> (84.7252, -33.8135)
  line L100 (72.8449, -38.6227) -> (77.6541, -33.8135)
  arc A145 (84.7252, -33.8135) -> (77.6541, -33.8135) centre (81.1896, -37.349) ccw
  line L101 (38.6227, -72.8449) -> (38.5865, -72.8811)
  line L102 (33.8327, -77.6349) -> (33.8316, -77.636)
  line L103 (38.6227, -72.8449) -> (33.8139, -77.6537)
  line L104 (35.2277, -86.1394) -> (33.8135, -84.7252)
  line L105 (33.8135, -84.7252) -> (33.7586, -84.6686)
  arc A146 (33.8139, -77.6537) -> (33.7586, -84.6686) centre (37.3495, -81.1892) ccw
  arc A147 (72.8811, 38.5865) -> (65.8101, 38.5865) centre (69.3456, 35.0509) ccw
  line L106 (-38.6227, 72.8449) -> (-33.8316, 77.636)
  line L107 (88.0068, -37.0951) -> (84.7252, -33.8135)
  arc A148 (-38.2288, -65.4524) -> (-38.6046, -72.863) centre (-35.0691, -69.3275) ccw
  line L108 (-72.863, 38.6046) -> (-38.5865, 72.8811)
  arc A149 (77.6349, 33.8327) -> (84.7081, 33.8327) centre (81.1715, 37.3672) ccw
  line L109 (-38.9441, -66.1678) -> (-15.8059, -43.0296)
  line L110 (-88.0068, 37.0951) -> (-84.7252, 33.8135)
  arc A150 (-62.2927, 49.1749) -> (-61.9168, 41.7643) centre (-58.7571, 45.6394) ccw
  arc A151 (-84.7263, 33.8146) -> (-77.653, 33.8146) centre (-81.1896, 37.349) ccw
  line L111 (38.9441, 66.1678) -> (15.8059, 43.0296)
  arc A152 (-42.122, 62.2745) -> (-49.1931, 62.2745) centre (-45.6575, 58.739) ccw
  arc A153 (33.8146, 84.7263) -> (33.8146, 77.653) centre (37.349, 81.1896) ccw
  arc A154 (38.2288, 65.4524) -> (38.6046, 72.863) centre (35.0691, 69.3275) ccw
  line L112 (65.8101, 38.5865) -> (43.0296, 15.8059)
  line L113 (-62.6322, 42.4797) -> (-43.4926, 23.3401)
  line L114 (38.6046, 72.863) -> (72.8811, 38.5865)